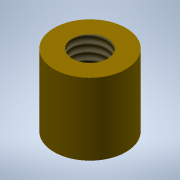
# Autodesk Inventor part: stand M3-L5
Saved by Autodesk Inventor 2022.6 (Build 266554000, 554)
## iProperties
Created: 2014-08-06
Part Number: stand M3-L5
Material: Generic
Document SubType Name: Modeling
Designer: s41607
Density: 1 g/cm^3
Appearance: Gold
Mass: 0.148859 g
Surface Area: 2.64103 cm^2
Volume: 0.148859 cm^3
Description: M3, 20mm stand
Author: s41607
Autodesk Inventor part; units mm, degrees
ref_plane "YZ Plane" through (0, 0, 0) normal (1, 0, 0) x (0, 1, 0)
ref_plane "XZ Plane" through (0, 0, 0) normal (0, 1, 0) x (-1, 0, 0)
ref_plane "XY Plane" through (0, 0, 0) normal (0, 0, 1) x (1, 0, 0)
sketch "Sketch1" plane through (0, 0, 0) normal (0, 0, 1) x (1, 0, 0)
  line L0 (-3.5, 0) -> (3.5, 0) projected
  line L1 (0, 3.5) -> (0, -3.5) projected
  circle A0 centre (0, 0) radius 2.5
  dimension "d0" = 5
  constraints: 1 centre point, 1 coincident
  measures "d0" diameter of A0
extrude "Extrusion1" add sketch "Sketch1" along normal blind 5
sketch "Sketch2" plane through (0, 0, 0) normal (0, 0, 1) x (1, 0, 0)
  line L0 (-14, 0) -> (14, 0) projected
  line L1 (0, 14) -> (0, -14) projected
  point P0 (0, 0)
  point P1 (0, 0)
  constraints: 1 coincident
hole "Hole1" at (0, 0, 0) direction (0, 0, 1) diameter 2.459 end through all thread size "M3x0.5" class "6H" standard "ISO Metric profile"
body "Solid1"
